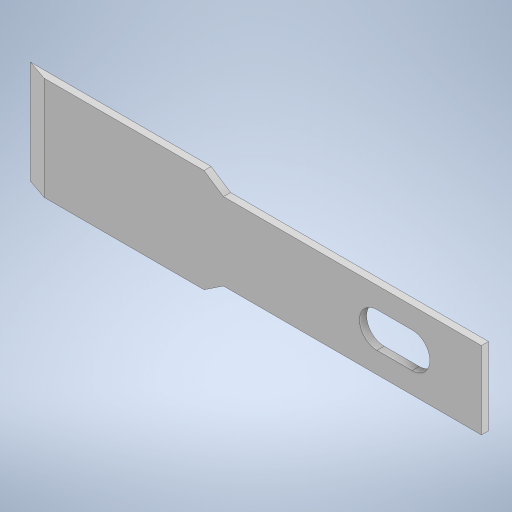
# Autodesk Inventor part: pen_type_cutter
Saved by Autodesk Inventor 2024.3 (Build 283343000, 343)
## iProperties
Created: 2025-06-07
Part Number: pen_type_cutter
Material: 一般
Document SubType Name: Modeling
Designer: hikou
Density: 1 g/cm^3
Appearance: 既定
Author: hikou
Autodesk Inventor part; units mm, degrees
ref_plane "YZ Plane" through (0, 0, 0) normal (1, 0, 0) x (0, 1, 0)
ref_plane "XZ Plane" through (0, 0, 0) normal (0, 1, 0) x (-1, 0, 0)
ref_plane "XY Plane" through (0, 0, 0) normal (0, 0, 1) x (1, 0, 0)
sketch "スケッチ1" plane through (0, 0, 0) normal (0, 0, 1) x (1, 0, 0)
  line L0 (-17.75, 4) -> (17.75, 4)
  line L1 (17.75, 4) -> (17.75, -4)
  line L2 (17.75, -4) -> (-17.75, -4)
  line L3 (-17.75, -4) -> (-17.75, 4)
  line L4 (-17.75, 4) -> (17.75, -4) construction
  line L5 (17.75, 4) -> (-17.75, -4) construction
  point P0 (0, 0)
  dimension "d0" = 35.5
  dimension "d1" = 8
  constraints: 12 end point, 2 midpoint, 2 parallel, 1 horizontal, 1 perpendicular
  measures "d0" distance of L1.end L2.end
  measures "d1" distance of L0.end L1.end
extrude "押し出し1" add sketch "スケッチ1" along normal mid plane 0.55
sketch "スケッチ2" plane through (0, 0, 0.275) normal (0, 0, 1) x (1, 0, 0)
  line L0 (9.6635, 0) -> (12.3865, 0) construction
  line L1 (9.6635, 1.3635) -> (12.3865, 1.3635)
  line L2 (12.3865, -1.3635) -> (9.6635, -1.3635)
  arc A0 (9.6635, 1.3635) -> (9.6635, -1.3635) centre (9.6635, 0) ccw
  arc A1 (12.3865, -1.3635) -> (12.3865, 1.3635) centre (12.3865, 0) ccw
  line L3 (17.75, -4) -> (17.75, 4) projected
  line L4 (17.75, 4) -> (-17.75, 4) projected
  point P0 (0, 0)
  point P1 (11.025, 0)
  point P2 (13.75, 0)
  point P3 (8.3, 0)
  dimension "d4" = 2.727
  dimension "d5" = 5.45
  dimension "d6" = 4
  dimension "d7" = 4
  constraints: 8 end point, 6 point on circle, 4 tangent, 2 centre point, 1 horizontal, 1 midpoint, 1 parallel
  measures "d4" distance between parallel lines of L2 L1
  measures "d5" distance of point (13.75, 0) point (8.3, 0)
  measures "d6" distance from line of L3 point (13.75, 0)
  measures "d7" distance between parallel lines of L4 L0
extrude "押し出し2" cut sketch "スケッチ2" against normal blind 0.55
sketch "スケッチ3" plane through (0, 0, 0.275) normal (0, 0, 1) x (1, 0, 0)
  line L0 (-17.75, 4) -> (17.75, 4) projected
  line L1 (17.75, 4) -> (17.75, -4) projected
  line L2 (-17.75, 4) -> (-17.75, -4) projected
  line L3 (-2.25, 3) -> (17.75, 3)
  line L4 (-3.75, 4) -> (-2.25, 3)
  line L5 (0, 0) -> (-1.8887, 0)
  line L6 (-2.25, -3) -> (17.75, -3)
  line L7 (-3.75, -4) -> (-2.25, -3)
  arc A0 (9.6635, 1.3635) -> (9.6635, -1.3635) centre (9.6635, 0) ccw projected
  line L8 (9.6635, 1.3635) -> (12.3865, 1.3635) projected
  arc A1 (12.3865, -1.3635) -> (12.3865, 1.3635) centre (12.3865, 0) ccw projected
  line L9 (12.3865, -1.3635) -> (9.6635, -1.3635) projected
  line L10 (-17.75, -4) -> (17.75, -4) projected
  line L11 (17.75, -4) -> (17.75, 4) projected
  line L12 (17.75, 4) -> (-17.75, 4) projected
  line L13 (-17.75, 4) -> (-17.75, -4) projected
  dimension "d10" = 1
  dimension "d11" = 14
  dimension "d12" = 20
  constraints: 10 end point, 3 symmetric about line, 2 point on line, 1 horizontal, 1 parallel
  measures "d10" distance from line of L0 L3.end
  measures "d11" distance from line of L2 L4.start
  measures "d12" distance of L3.end L3.start
extrude "押し出し3" cut sketch "スケッチ3" against normal blind 0.55 contours L0 L1 L3 L4 | L7 L6 L1 L10
sketch "スケッチ4" plane through (-17.75, -4, -0.275) normal (0, -1, 0) x (1, 0, 0)
  line L0 (0, 0.55) -> (14, 0.55) projected
  line L1 (0, 0.55) -> (0, 0) projected
  line L2 (0, 0) -> (1.6, 0.55)
  point P0 (17.75, 0.275)
  dimension "d15" = 1.6
  constraints: 2 end point, 1 point on line
  measures "d15" distance of L2.end L0.start
extrude "押し出し4" cut sketch "スケッチ4" against normal through all
